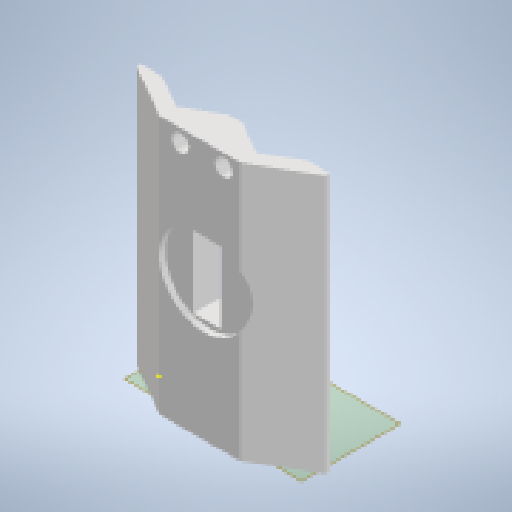
# Autodesk Inventor part: крепеж бок
Saved by Autodesk Inventor 2024.2 (Build 282272000, 272)
## iProperties
Created: 2026-04-23
Part Number: крепеж бок
Material: Типовые
Document SubType Name: Modeling
Designer: katya_notebook
Density: 1 g/cm^3
Appearance: По умолчанию
Author: katya_notebook
Autodesk Inventor part; units mm, degrees
ref_plane "YZ Plane" through (0, 0, 0) normal (1, 0, 0) x (0, 1, 0)
ref_plane "XZ Plane" through (0, 0, 0) normal (0, 1, 0) x (-1, 0, 0)
ref_plane "РабПлоскость1" through (19.6, -8, -11) normal (0, -1, 0) x (-1, 0, 0)
sketch "Эскиз1" plane through (19.6, -8, -11) normal (0, -1, 0) x (-1, 0, 0)
  line L0 (29.4, -5.9741) -> (29.4, 5.9741) projected
  line L1 (28.2551, 5.9741) -> (29.4, 5.9741) projected
  line L2 (28.65, 6.658) -> (28.2551, 5.9741) projected
  line L3 (27.6679, 6.658) -> (28.65, 6.658) projected
  line L4 (21.3321, 10.3161) -> (27.6679, 6.658) projected
  line L5 (21.3321, 10.3161) -> (20.35, 10.3161) projected
  line L6 (20.35, 10.3161) -> (20.5955, 10.7413) projected
  line L7 (20.1474, 11) -> (20.5955, 10.7413) projected
  line L8 (20.1474, 11) -> (19.0526, 11) projected
  line L9 (18.6045, 10.7413) -> (19.0526, 11) projected
  line L10 (18.85, 10.3161) -> (18.6045, 10.7413) projected
  line L11 (17.8679, 10.3161) -> (18.85, 10.3161) projected
  line L12 (11.5321, 6.658) -> (17.8679, 10.3161) projected
  line L13 (11.5321, 6.658) -> (10.55, 6.658) projected
  line L14 (10.55, 6.658) -> (10.9449, 5.9741) projected
  line L15 (8.6551, 5.9741) -> (10.9449, 5.9741) projected
  line L16 (9.05, 6.658) -> (8.6551, 5.9741) projected
  line L17 (8.0679, 6.658) -> (9.05, 6.658) projected
  line L18 (1.7321, 10.3161) -> (8.0679, 6.658) projected
  line L19 (1.7321, 10.3161) -> (0.75, 10.3161) projected
  line L20 (0.75, 10.3161) -> (0.9955, 10.7413) projected
  line L21 (0.5474, 11) -> (0.9955, 10.7413) projected
  line L22 (-0.5474, 11) -> (0.5474, 11) projected
  line L23 (-0.9955, 10.7413) -> (-0.5474, 11) projected
  line L24 (-0.75, 10.3161) -> (-0.9955, 10.7413) projected
  line L25 (-1.7321, 10.3161) -> (-0.75, 10.3161) projected
  line L26 (-8.0679, 6.658) -> (-1.7321, 10.3161) projected
  line L27 (-8.0679, 6.658) -> (-9.05, 6.658) projected
  line L28 (-9.05, 6.658) -> (-8.6551, 5.9741) projected
  line L29 (-8.6551, 5.9741) -> (-9.8, 5.9741) projected
  line L30 (-9.8, -5.9741) -> (-9.8, 5.9741) projected
  line L31 (-8.6551, -5.9741) -> (-9.8, -5.9741) projected
  line L32 (-9.05, -6.658) -> (-8.6551, -5.9741) projected
  line L33 (-8.0679, -6.658) -> (-9.05, -6.658) projected
  line L34 (-1.7321, -10.3161) -> (-8.0679, -6.658) projected
  line L35 (-1.7321, -10.3161) -> (-0.75, -10.3161) projected
  line L36 (-0.75, -10.3161) -> (-0.9955, -10.7413) projected
  line L37 (-0.5474, -11) -> (-0.9955, -10.7413) projected
  line L38 (-0.5474, -11) -> (0.5474, -11) projected
  line L39 (0.9955, -10.7413) -> (0.5474, -11) projected
  line L40 (0.75, -10.3161) -> (0.9955, -10.7413) projected
  line L41 (1.7321, -10.3161) -> (0.75, -10.3161) projected
  line L42 (8.0679, -6.658) -> (1.7321, -10.3161) projected
  line L43 (8.0679, -6.658) -> (9.05, -6.658) projected
  line L44 (9.05, -6.658) -> (8.6551, -5.9741) projected
  line L45 (8.6551, -5.9741) -> (10.9449, -5.9741) projected
  line L46 (10.55, -6.658) -> (10.9449, -5.9741) projected
  line L47 (11.5321, -6.658) -> (10.55, -6.658) projected
  line L48 (17.8679, -10.3161) -> (11.5321, -6.658) projected
  line L49 (17.8679, -10.3161) -> (18.85, -10.3161) projected
  line L50 (18.85, -10.3161) -> (18.6045, -10.7413) projected
  line L51 (19.0526, -11) -> (18.6045, -10.7413) projected
  line L52 (19.0526, -11) -> (20.1474, -11) projected
  line L53 (20.5955, -10.7413) -> (20.1474, -11) projected
  line L54 (20.35, -10.3161) -> (20.5955, -10.7413) projected
  line L55 (21.3321, -10.3161) -> (20.35, -10.3161) projected
  line L56 (27.6679, -6.658) -> (21.3321, -10.3161) projected
  line L57 (27.6679, -6.658) -> (28.65, -6.658) projected
  line L58 (28.65, -6.658) -> (28.2551, -5.9741) projected
  line L59 (28.2551, -5.9741) -> (29.4, -5.9741) projected
  circle A0 centre (0, 0) radius 8.1 projected
  circle A1 centre (19.6, 0) radius 8.1 projected
  line L60 (32.9, 3.6373) -> (42.7, 9.2953) projected
  line L61 (42.7, 9.2953) -> (42.7, 24.6529) projected
  line L62 (42.7, 24.6529) -> (29.4, 32.3316) projected
  line L63 (29.4, 32.3316) -> (19.6, 26.6736) projected
  line L64 (19.6, 26.6736) -> (9.8, 32.3316) projected
  line L65 (9.8, 32.3316) -> (0, 26.6736) projected
  line L66 (0, 26.6736) -> (-9.8, 32.3316) projected
  line L67 (-9.8, 32.3316) -> (-23.1, 24.6529) projected
  line L68 (-23.1, 24.6529) -> (-23.1, 9.2953) projected
  line L69 (-23.1, 9.2953) -> (-13.3, 3.6373) projected
  line L70 (-13.3, 3.6373) -> (-13.3, -7.6788) projected
  line L71 (29.4, -5.9741) -> (28.2551, -5.9741) projected
  line L72 (28.2551, -5.9741) -> (28.65, -6.658) projected
  line L73 (28.65, -6.658) -> (27.6679, -6.658) projected
  line L74 (27.6679, -6.658) -> (21.3321, -10.3161) projected
  line L75 (17.8679, -10.3161) -> (11.5321, -6.658) projected
  line L76 (11.5321, -6.658) -> (10.55, -6.658) projected
  line L77 (10.55, -6.658) -> (10.9449, -5.9741) projected
  line L78 (10.9449, -5.9741) -> (8.6551, -5.9741) projected
  line L79 (8.6551, -5.9741) -> (9.05, -6.658) projected
  line L80 (9.05, -6.658) -> (8.0679, -6.658) projected
  line L81 (8.0679, -6.658) -> (1.7321, -10.3161) projected
  line L82 (-1.7321, -10.3161) -> (-8.0679, -6.658) projected
  line L83 (-8.0679, -6.658) -> (-9.05, -6.658) projected
  line L84 (-9.05, -6.658) -> (-8.6551, -5.9741) projected
  line L85 (-8.6551, -5.9741) -> (-9.8, -5.9741) projected
  line L86 (-9.8, -5.9741) -> (-9.8, 5.9741) projected
  line L87 (-9.8, 5.9741) -> (-10.3474, 5.9741) projected
  line L88 (-10.3474, 5.9741) -> (-10.7955, 6.2328) projected
  line L89 (-10.7955, 6.2328) -> (-10.55, 6.658) projected
  line L90 (-10.55, 6.658) -> (-11.5321, 6.658) projected
  line L91 (-11.5321, 6.658) -> (-17.8679, 10.3161) projected
  line L92 (-17.8679, 10.3161) -> (-18.85, 10.3161) projected
  line L93 (-18.85, 10.3161) -> (-18.4551, 11) projected
  line L94 (-18.4551, 11) -> (-19.6, 11) projected
  line L95 (-19.6, 11) -> (-19.6, 22.9482) projected
  line L96 (-19.6, 22.9482) -> (-18.4551, 22.9482) projected
  line L97 (-18.4551, 22.9482) -> (-18.85, 23.6321) projected
  line L98 (-18.85, 23.6321) -> (-17.8679, 23.6321) projected
  line L99 (-17.8679, 23.6321) -> (-11.5321, 27.2902) projected
  line L100 (-11.5321, 27.2902) -> (-10.55, 27.2902) projected
  line L101 (-10.55, 27.2902) -> (-10.7955, 27.7154) projected
  line L102 (-10.7955, 27.7154) -> (-10.3474, 27.9741) projected
  line L103 (-10.3474, 27.9741) -> (-9.2526, 27.9741) projected
  line L104 (-9.2526, 27.9741) -> (-8.8045, 27.7154) projected
  line L105 (-8.8045, 27.7154) -> (-9.05, 27.2902) projected
  line L106 (-9.05, 27.2902) -> (-8.0679, 27.2902) projected
  line L107 (-8.0679, 27.2902) -> (-1.7321, 23.6321) projected
  line L108 (-1.7321, 23.6321) -> (-0.75, 23.6321) projected
  line L109 (-0.75, 23.6321) -> (-1.1449, 22.9482) projected
  line L110 (-1.1449, 22.9482) -> (1.1449, 22.9482) projected
  line L111 (1.1449, 22.9482) -> (0.75, 23.6321) projected
  line L112 (0.75, 23.6321) -> (1.7321, 23.6321) projected
  line L113 (1.7321, 23.6321) -> (8.0679, 27.2902) projected
  line L114 (8.0679, 27.2902) -> (9.05, 27.2902) projected
  line L115 (9.05, 27.2902) -> (8.8045, 27.7154) projected
  line L116 (8.8045, 27.7154) -> (9.2526, 27.9741) projected
  line L117 (9.2526, 27.9741) -> (10.3474, 27.9741) projected
  line L118 (10.3474, 27.9741) -> (10.7955, 27.7154) projected
  line L119 (10.7955, 27.7154) -> (10.55, 27.2902) projected
  line L120 (10.55, 27.2902) -> (11.5321, 27.2902) projected
  line L121 (11.5321, 27.2902) -> (17.8679, 23.6321) projected
  line L122 (17.8679, 23.6321) -> (18.85, 23.6321) projected
  line L123 (18.85, 23.6321) -> (18.4551, 22.9482) projected
  line L124 (18.4551, 22.9482) -> (20.7449, 22.9482) projected
  line L125 (20.7449, 22.9482) -> (20.35, 23.6321) projected
  line L126 (20.35, 23.6321) -> (21.3321, 23.6321) projected
  line L127 (21.3321, 23.6321) -> (27.6679, 27.2902) projected
  line L128 (27.6679, 27.2902) -> (28.65, 27.2902) projected
  line L129 (28.65, 27.2902) -> (28.4045, 27.7154) projected
  line L130 (28.4045, 27.7154) -> (28.8526, 27.9741) projected
  line L131 (28.8526, 27.9741) -> (29.9474, 27.9741) projected
  line L132 (29.9474, 27.9741) -> (30.3955, 27.7154) projected
  line L133 (30.3955, 27.7154) -> (30.15, 27.2902) projected
  line L134 (30.15, 27.2902) -> (31.1321, 27.2902) projected
  line L135 (31.1321, 27.2902) -> (37.4679, 23.6321) projected
  line L136 (37.4679, 23.6321) -> (38.45, 23.6321) projected
  line L137 (38.45, 23.6321) -> (38.0551, 22.9482) projected
  line L138 (38.0551, 22.9482) -> (39.2, 22.9482) projected
  line L139 (39.2, 22.9482) -> (39.2, 11) projected
  line L140 (39.2, 11) -> (38.0551, 11) projected
  line L141 (38.0551, 11) -> (38.45, 10.3161) projected
  line L142 (38.45, 10.3161) -> (37.4679, 10.3161) projected
  line L143 (37.4679, 10.3161) -> (31.1321, 6.658) projected
  line L144 (31.1321, 6.658) -> (30.15, 6.658) projected
  line L145 (30.15, 6.658) -> (30.3955, 6.2328) projected
  line L146 (30.3955, 6.2328) -> (29.9474, 5.9741) projected
  line L147 (29.9474, 5.9741) -> (29.4, 5.9741) projected
  line L148 (29.4, 5.9741) -> (29.4, -5.9741) projected
  line L149 (-13.3, -7.6788) -> (0, -15.3575) projected
  line L150 (0, -15.3575) -> (9.8, -9.6995) projected
  line L151 (9.8, -9.6995) -> (19.6, -15.3575) projected
  line L152 (19.6, -15.3575) -> (32.9, -7.6788) projected
  line L153 (32.9, -7.6788) -> (32.9, 3.6373) projected
  line L154 (21.3321, -10.3161) -> (20.35, -10.3161) projected
  line L155 (20.35, -10.3161) -> (20.5955, -10.7413) projected
  line L156 (20.5955, -10.7413) -> (20.1474, -11) projected
  line L157 (20.1474, -11) -> (19.0526, -11) projected
  line L158 (19.0526, -11) -> (18.6045, -10.7413) projected
  line L159 (18.6045, -10.7413) -> (18.85, -10.3161) projected
  line L160 (18.85, -10.3161) -> (17.8679, -10.3161) projected
  line L161 (1.7321, -10.3161) -> (0.75, -10.3161) projected
  line L162 (0.75, -10.3161) -> (0.9955, -10.7413) projected
  line L163 (0.9955, -10.7413) -> (0.5474, -11) projected
  line L164 (0.5474, -11) -> (-0.5474, -11) projected
  line L165 (-0.5474, -11) -> (-0.9955, -10.7413) projected
  line L166 (-0.9955, -10.7413) -> (-0.75, -10.3161) projected
  line L167 (-0.75, -10.3161) -> (-1.7321, -10.3161) projected
  line L168 (32.9, -5.9741) -> (29.4, -5.9741)
  line L169 (-9.8, -5.9741) -> (-13.3, -5.9741)
  line L170 (19.6, -15.3575) -> (0, -15.3575)
  point P0 (19.6, -11)
  constraints: 6 end point, 2 perpendicular, 2 point on line, 1 horizontal
ref_plane "РабПлоскость2" through (-38.0502, 55.1, -60.2624) normal (0, -1, 0) x (1, 0, 0)
extrude "Выдавливание1" add sketch "Эскиз1" against normal up to surface (63.1 mm away) contours L168 L153 L152 L151 L150 L149 L70 L169 L31 L32 L33 L34 L35 L36 L37 L38 L39 L40 L41 L42 L43 L44 L45 L46 L47 L48 L49 L50 L51 L52 L53 L54 L55 L56 L57 L58 L59 | L170 L150 L151
sketch "Эскиз2" plane through (0, -8, 4.3575) normal (0, 0, 1) x (1, 0, 0)
  circle A0 centre (10.0964, 32.8819) radius 10.85 projected
  spline S0 degree 3 poles (1.2199, 29.8332) (1.2264, 29.8391) (1.2399, 29.8514) (1.2666, 29.8618) (1.2971, 29.8679) (1.3188, 29.8674) (1.3303, 29.8671) knots 0 0 0 0 0.219432 0.455746 0.710361 1 1 1 1 projected
  line L0 (1.3303, 29.8671) -> (4.8998, 29.6603) projected
  line L1 (4.8998, 29.6603) -> (4.9412, 30.3747) projected
  spline S1 degree 3 poles (4.9412, 30.3747) (4.9436, 30.3952) (4.948, 30.4343) (4.9731, 30.4645) (4.9851, 30.4789) knots 0 0 0 0 0.523055 1 1 1 1 projected
  spline S2 degree 3 poles (4.9851, 30.4789) (5.0002, 30.4888) (5.0301, 30.5084) (5.0658, 30.5096) (5.0835, 30.5102) knots 0 0 0 0 0.505194 1 1 1 1 projected
  spline S3 degree 3 poles (5.0835, 30.5102) (5.0953, 30.507) (5.1242, 30.4991) (5.1574, 30.4755) (5.186, 30.4505) (5.2006, 30.4236) (5.2097, 30.3936) (5.2095, 30.3722) (5.2093, 30.3609) knots 0 0 0 0 0.170693 0.418909 0.563896 0.700202 0.841955 1 1 1 1 projected
  line L2 (5.2093, 30.3609) -> (5.1108, 28.6607) projected
  spline S4 degree 3 poles (5.1108, 28.6607) (5.1075, 28.6439) (5.1004, 28.6081) (5.064, 28.5657) (5.0204, 28.5312) (4.985, 28.5283) (4.9686, 28.5269) knots 0 0 0 0 0.239185 0.507115 0.772399 1 1 1 1 projected
  spline S5 degree 3 poles (4.9686, 28.5269) (4.9527, 28.5298) (4.9195, 28.5357) (4.8843, 28.5622) (4.8611, 28.5897) (4.8491, 28.6156) (4.842, 28.6452) (4.8426, 28.6661) (4.8429, 28.6771) knots 0 0 0 0 0.219722 0.460095 0.585443 0.71296 0.849405 1 1 1 1 projected
  line L3 (4.8429, 28.6771) -> (4.8843, 29.3923) projected
  line L4 (4.8843, 29.3923) -> (1.3148, 29.5991) projected
  spline S6 degree 3 poles (1.3148, 29.5991) (1.2937, 29.6014) (1.254, 29.6057) (1.2233, 29.6311) (1.2089, 29.6431) knots 0 0 0 0 0.529822 1 1 1 1 projected
  spline S7 degree 3 poles (1.2089, 29.6431) (1.1996, 29.6574) (1.1802, 29.6872) (1.1802, 29.7228) (1.1802, 29.7414) knots 0 0 0 0 0.479535 1 1 1 1 projected
  spline S8 degree 3 poles (1.1802, 29.7414) (1.1812, 29.7464) (1.1836, 29.7582) (1.1913, 29.7787) (1.2037, 29.8042) (1.2142, 29.8229) (1.2199, 29.8332) knots 0 0 0 0 0.152278 0.360896 0.649123 1 1 1 1 projected
  line L5 (5.314, 32.1682) -> (5.2899, 31.752) projected
  spline S9 degree 3 poles (5.2899, 31.752) (5.2876, 31.7272) (5.2829, 31.6758) (5.2703, 31.5966) (5.2484, 31.514) (5.2231, 31.428) (5.1921, 31.3426) (5.1551, 31.2607) (5.1134, 31.1842) (5.0808, 31.137) (5.0647, 31.1138) knots 0 0 0 0 0.109156 0.226197 0.350912 0.483159 0.618823 0.74875 0.876439 1 1 1 1 projected
  spline S10 degree 3 poles (5.0647, 31.1138) (5.0604, 31.1082) (5.0508, 31.0957) (5.0277, 31.0797) (4.9933, 31.0643) (4.9651, 31.0584) (4.9487, 31.055) knots 0 0 0 0 0.157275 0.353812 0.623959 1 1 1 1 projected
  spline S11 degree 3 poles (4.9487, 31.055) (4.931, 31.0577) (4.8944, 31.0635) (4.8502, 31.0969) (4.8148, 31.1372) (4.811, 31.1704) (4.8092, 31.1857) knots 0 0 0 0 0.254223 0.52772 0.782584 1 1 1 1 projected
  line L6 (4.8092, 31.1857) -> (4.839, 31.2655) projected
  spline S12 degree 3 poles (4.839, 31.2655) (4.8649, 31.302) (4.9161, 31.3743) (4.9704, 31.4963) (5.009, 31.625) (5.0173, 31.7147) (5.0215, 31.76) knots 0 0 0 0 0.250207 0.496054 0.745305 1 1 1 1 projected
  line L7 (5.0215, 31.76) -> (5.0462, 32.1871) projected
  spline S13 degree 3 poles (5.0462, 32.1871) (5.0465, 32.2279) (5.047, 32.3069) (5.0221, 32.4217) (4.9727, 32.5253) (4.9041, 32.6172) (4.8204, 32.6936) (4.7258, 32.7518) (4.6219, 32.7904) (4.5485, 32.7982) (4.5113, 32.8021) knots 0 0 0 0 0.134588 0.260434 0.384536 0.51119 0.637382 0.756913 0.876544 1 1 1 1 projected
  line L8 (4.5113, 32.8021) -> (4.3969, 32.8004) projected
  line L9 (4.3969, 32.8004) -> (4.3418, 32.7918) projected
  line L10 (4.3418, 32.7918) -> (4.2895, 32.7747) projected
  spline S14 degree 3 poles (4.2895, 32.7747) (4.2759, 32.7681) (4.2464, 32.7539) (4.201, 32.7264) (4.1502, 32.6923) (4.1153, 32.6662) (4.0967, 32.6522) knots 0 0 0 0 0.198705 0.428492 0.695375 1 1 1 1 projected
  line L11 (4.0967, 32.6522) -> (2.7508, 31.4386) projected
  spline S15 degree 3 poles (2.7508, 31.4386) (2.7287, 31.4196) (2.6853, 31.3821) (2.6147, 31.3335) (2.5398, 31.2938) (2.4871, 31.2738) (2.4608, 31.2638) knots 0 0 0 0 0.25594 0.505009 0.752321 1 1 1 1 projected
  line L12 (2.4608, 31.2638) -> (2.3941, 31.2441) projected
  line L13 (2.3941, 31.2441) -> (2.2844, 31.2219) projected
  line L14 (2.2844, 31.2219) -> (2.2184, 31.214) projected
  line L15 (2.2184, 31.214) -> (2.1355, 31.2188) projected
  spline S16 degree 3 poles (2.1355, 31.2188) (2.1073, 31.221) (2.0518, 31.2253) (1.9706, 31.2414) (1.8929, 31.264) (1.8193, 31.2949) (1.7487, 31.3318) (1.6814, 31.3759) (1.6185, 31.428) (1.5798, 31.4669) (1.5603, 31.4866) knots 0 0 0 0 0.130274 0.256409 0.380833 0.502298 0.624003 0.747576 0.872087 1 1 1 1 projected
  spline S17 degree 3 poles (1.5603, 31.4866) (1.5403, 31.5086) (1.501, 31.552) (1.4514, 31.6239) (1.409, 31.6982) (1.3765, 31.777) (1.3515, 31.8588) (1.3368, 31.9447) (1.3286, 32.0337) (1.3307, 32.0942) (1.3317, 32.125) knots 0 0 0 0 0.127376 0.251339 0.373922 0.494219 0.616919 0.74041 0.867775 1 1 1 1 projected
  line L16 (1.3317, 32.125) -> (1.3558, 32.5404) projected
  spline S18 degree 3 poles (1.3558, 32.5404) (1.3581, 32.57) (1.3627, 32.6288) (1.3785, 32.7152) (1.3986, 32.7994) (1.4276, 32.8801) (1.4612, 32.9589) (1.503, 33.0341) (1.5498, 33.1077) (1.5861, 33.1534) (1.6044, 33.1765) knots 0 0 0 0 0.128087 0.254502 0.3786 0.501671 0.623923 0.748156 0.873068 1 1 1 1 projected
  line L17 (1.6044, 33.1765) -> (1.6608, 33.2219) projected
  line L18 (1.6608, 33.2219) -> (1.7278, 33.2323) projected
  spline S19 degree 3 poles (1.7278, 33.2323) (1.7436, 33.2293) (1.7788, 33.2226) (1.8172, 33.1955) (1.8457, 33.1692) (1.862, 33.1468) (1.8715, 33.123) (1.872, 33.1067) (1.8722, 33.0988) knots 0 0 0 0 0.225013 0.500357 0.645758 0.771988 0.888482 1 1 1 1 projected
  line L19 (1.8722, 33.0988) -> (1.8363, 33.0168) projected
  spline S20 degree 3 poles (1.8363, 33.0168) (1.8059, 32.9802) (1.7465, 32.909) (1.6822, 32.7873) (1.6385, 32.66) (1.6288, 32.5716) (1.6239, 32.5274) knots 0 0 0 0 0.262033 0.510647 0.755153 1 1 1 1 projected
  line L20 (1.6239, 32.5274) -> (1.5994, 32.1045) projected
  spline S21 degree 3 poles (1.5994, 32.1045) (1.5993, 32.0662) (1.5991, 31.9907) (1.6258, 31.8801) (1.6754, 31.7771) (1.7439, 31.6831) (1.827, 31.6017) (1.9225, 31.5408) (2.0268, 31.4999) (2.1004, 31.4917) (2.1376, 31.4876) knots 0 0 0 0 0.126552 0.249346 0.372878 0.503227 0.632635 0.755805 0.876214 1 1 1 1 projected
  line L21 (2.1376, 31.4876) -> (2.2344, 31.4904) projected
  spline S22 degree 3 poles (2.2344, 31.4904) (2.2424, 31.4911) (2.2593, 31.4927) (2.2852, 31.4995) (2.3126, 31.5062) (2.3305, 31.5129) (2.3393, 31.5162) knots 0 0 0 0 0.220277 0.47027 0.739664 1 1 1 1 projected
  spline S23 degree 3 poles (2.3393, 31.5162) (2.3561, 31.5216) (2.3912, 31.5327) (2.4427, 31.5592) (2.4967, 31.5921) (2.5308, 31.6198) (2.5487, 31.6344) knots 0 0 0 0 0.217508 0.45648 0.715095 1 1 1 1 projected
  line L22 (2.5487, 31.6344) -> (3.8947, 32.8496) projected
  spline S24 degree 3 poles (3.8947, 32.8496) (3.9135, 32.8658) (3.9528, 32.8998) (4.0224, 32.9431) (4.0991, 32.9892) (4.1556, 33.0157) (4.1849, 33.0295) knots 0 0 0 0 0.216591 0.454587 0.716038 1 1 1 1 projected
  spline S25 degree 3 poles (4.1849, 33.0295) (4.2113, 33.037) (4.2639, 33.0522) (4.3449, 33.067) (4.4272, 33.0731) (4.4823, 33.0718) (4.5101, 33.0711) knots 0 0 0 0 0.249589 0.498449 0.747622 1 1 1 1 projected
  spline S26 degree 3 poles (4.5101, 33.0711) (4.5383, 33.0689) (4.5938, 33.0646) (4.675, 33.0485) (4.7526, 33.0259) (4.8263, 32.995) (4.8966, 32.958) (4.9644, 32.915) (5.0271, 32.8627) (5.0658, 32.8238) (5.0853, 32.8042) knots 0 0 0 0 0.130358 0.256573 0.381077 0.50262 0.624402 0.747414 0.872005 1 1 1 1 projected
  spline S27 degree 3 poles (5.0853, 32.8042) (5.1053, 32.7822) (5.1447, 32.7388) (5.1939, 32.667) (5.2369, 32.5933) (5.2689, 32.5147) (5.2944, 32.4334) (5.3089, 32.3477) (5.317, 32.259) (5.3151, 32.1988) (5.314, 32.1682) knots 0 0 0 0 0.127803 0.252181 0.37416 0.49486 0.61684 0.740744 0.868535 1 1 1 1 projected
  spline S28 degree 3 poles (3.6331, 34.2513) (3.6171, 34.2541) (3.5836, 34.26) (3.549, 34.2875) (3.5256, 34.3149) (3.5136, 34.3409) (3.5065, 34.3704) (3.5071, 34.3913) (3.5074, 34.4023) knots 0 0 0 0 0.219271 0.461203 0.586294 0.713549 0.849714 1 1 1 1 projected
  line L23 (3.5074, 34.4023) -> (3.5487, 35.1167) projected
  line L24 (3.5487, 35.1167) -> (1.7799, 35.2192) projected
  line L25 (1.7799, 35.2192) -> (1.7054, 33.9336) projected
  spline S29 degree 3 poles (1.7054, 33.9336) (1.7021, 33.9168) (1.695, 33.8811) (1.6586, 33.8386) (1.6149, 33.8043) (1.5795, 33.8007) (1.5632, 33.799) knots 0 0 0 0 0.238964 0.506645 0.771683 1 1 1 1 projected
  spline S30 degree 3 poles (1.5632, 33.799) (1.5473, 33.8019) (1.514, 33.8078) (1.4789, 33.8343) (1.4556, 33.8618) (1.4436, 33.8877) (1.4366, 33.917) (1.4371, 33.9376) (1.4374, 33.9483) knots 0 0 0 0 0.220569 0.461868 0.587699 0.715707 0.852678 1 1 1 1 projected
  line L26 (1.4374, 33.9483) -> (1.5192, 35.3612) projected
  spline S31 degree 3 poles (1.5192, 35.3612) (1.5219, 35.3821) (1.5267, 35.4202) (1.5572, 35.4694) (1.6096, 35.494) (1.6479, 35.4943) (1.669, 35.4946) knots 0 0 0 0 0.274617 0.5 0.725383 1 1 1 1 projected
  line L27 (1.669, 35.4946) -> (5.3524, 35.2811) projected
  spline S32 degree 3 poles (5.3524, 35.2811) (5.3733, 35.2785) (5.4113, 35.2737) (5.4605, 35.2432) (5.4851, 35.1908) (5.4855, 35.1525) (5.4857, 35.1314) knots 0 0 0 0 0.274617 0.5 0.725383 1 1 1 1 projected
  line L28 (5.4857, 35.1314) -> (5.4039, 33.7185) projected
  spline S33 degree 3 poles (5.4039, 33.7185) (5.4005, 33.7017) (5.3934, 33.6659) (5.3571, 33.6235) (5.3134, 33.589) (5.278, 33.5861) (5.2617, 33.5847) knots 0 0 0 0 0.239185 0.507115 0.772399 1 1 1 1 projected
  spline S34 degree 3 poles (5.2617, 33.5847) (5.2457, 33.5875) (5.2122, 33.5934) (5.1776, 33.6208) (5.1542, 33.6483) (5.1422, 33.6742) (5.1352, 33.7035) (5.1356, 33.7242) (5.1359, 33.7349) knots 0 0 0 0 0.220114 0.462976 0.588548 0.716293 0.852982 1 1 1 1 projected
  line L29 (5.1359, 33.7349) -> (5.2104, 35.0205) projected
  line L30 (5.2104, 35.0205) -> (3.8168, 35.1012) projected
  line L31 (3.8168, 35.1012) -> (3.7754, 34.3868) projected
  spline S35 degree 3 poles (3.7754, 34.3868) (3.772, 34.3697) (3.7651, 34.3336) (3.7285, 34.2909) (3.6848, 34.2566) (3.6494, 34.253) (3.6331, 34.2513) knots 0 0 0 0 0.241893 0.508544 0.772562 1 1 1 1 projected
  spline S36 degree 3 poles (1.6423, 37.123) (1.6488, 37.1289) (1.6622, 37.1412) (1.689, 37.1516) (1.7195, 37.1577) (1.7411, 37.1572) (1.7527, 37.1569) knots 0 0 0 0 0.219432 0.455746 0.710361 1 1 1 1 projected
  line L32 (1.7527, 37.1569) -> (5.3222, 36.9501) projected
  line L33 (5.3222, 36.9501) -> (5.3636, 37.6645) projected
  spline S37 degree 3 poles (5.3636, 37.6645) (5.3659, 37.685) (5.3704, 37.7241) (5.3955, 37.7543) (5.4074, 37.7687) knots 0 0 0 0 0.523055 1 1 1 1 projected
  spline S38 degree 3 poles (5.4074, 37.7687) (5.4225, 37.7786) (5.4525, 37.7982) (5.4882, 37.7994) (5.5059, 37.8) knots 0 0 0 0 0.505194 1 1 1 1 projected
  spline S39 degree 3 poles (5.5059, 37.8) (5.5177, 37.7967) (5.5466, 37.7889) (5.5798, 37.7652) (5.6084, 37.7402) (5.623, 37.7134) (5.6321, 37.6834) (5.6318, 37.662) (5.6317, 37.6507) knots 0 0 0 0 0.170693 0.418909 0.563896 0.700202 0.841955 1 1 1 1 projected
  line L34 (5.6317, 37.6507) -> (5.5332, 35.9505) projected
  spline S40 degree 3 poles (5.5332, 35.9505) (5.5298, 35.9336) (5.5228, 35.8979) (5.4864, 35.8555) (5.4427, 35.8209) (5.4073, 35.8181) (5.391, 35.8167) knots 0 0 0 0 0.239185 0.507115 0.772399 1 1 1 1 projected
  spline S41 degree 3 poles (5.391, 35.8167) (5.3751, 35.8196) (5.3418, 35.8255) (5.3067, 35.852) (5.2834, 35.8795) (5.2714, 35.9054) (5.2644, 35.935) (5.2649, 35.9559) (5.2652, 35.9669) knots 0 0 0 0 0.219722 0.460095 0.585443 0.71296 0.849405 1 1 1 1 projected
  line L35 (5.2652, 35.9669) -> (5.3067, 36.6821) projected
  line L36 (5.3067, 36.6821) -> (1.7371, 36.8889) projected
  spline S42 degree 3 poles (1.7371, 36.8889) (1.7161, 36.8912) (1.6764, 36.8955) (1.6457, 36.9209) (1.6313, 36.9329) knots 0 0 0 0 0.529822 1 1 1 1 projected
  spline S43 degree 3 poles (1.6313, 36.9329) (1.622, 36.9472) (1.6025, 36.977) (1.6025, 37.0126) (1.6025, 37.0312) knots 0 0 0 0 0.479535 1 1 1 1 projected
  spline S44 degree 3 poles (1.6025, 37.0312) (1.6035, 37.0362) (1.606, 37.048) (1.6136, 37.0685) (1.6261, 37.094) (1.6366, 37.1127) (1.6423, 37.123) knots 0 0 0 0 0.152278 0.360896 0.649123 1 1 1 1 projected
  arc A1 (13.962, 34.3771) -> (13.7634, 30.9503) centre (10.0964, 32.8819) ccw projected
  line L37 (13.962, 34.3771) -> (13.2158, 34.0885) projected
  arc A2 (13.2158, 34.0885) -> (13.0556, 31.3231) centre (10.0964, 32.8819) ccw projected
  line L38 (13.0556, 31.3231) -> (13.7634, 30.9503) projected
  line L39 (14.9235, 33.0029) -> (12.2087, 33.1602) projected
  line L40 (14.9235, 33.0029) -> (14.8772, 32.2042) projected
  line L41 (14.8772, 32.2042) -> (12.1624, 32.3615) projected
  line L42 (12.1624, 32.3615) -> (12.2087, 33.1602) projected
  line L43 (13.5198, 41.5398) -> (6.7574, 41.5398)
  line L44 (6.7574, 41.5398) -> (6.7574, 24.0382)
  line L45 (6.7574, 24.0382) -> (13.5198, 24.0382)
  line L46 (13.5198, 24.0382) -> (13.5198, 41.5398)
  point P0 (0, 8)
  constraints: 8 end point, 2 parallel, 1 horizontal, 1 perpendicular
extrude "Выдавливание2" cut sketch "Эскиз2" against normal blind 10 contours L46 L37 A2 L44 A1 | A1 L44 L43 L46 | L46 L39 L42 L41 L38 A2 L44 L37 | L46 L41 L42 L39 | L44 A2 L38 L46 A1 | A1 L46 L45 L44
sketch "Эскиз3" plane through (0, -8, 4.3575) normal (0, 0, 1) x (1, 0, 0)
  circle A0 centre (10.8015, 33.6616) radius 10.85 projected
  point P0 (0, 8)
extrude "Выдавливание3" cut sketch "Эскиз3" against normal blind 1.5
sketch "Эскиз4" plane through (0, 55.1, 4.3575) normal (0, 0, 1) x (1, 0, 0)
  point P0 (0, -55.1)
sketch "Эскиз5" plane through (0, 55.1, 4.3575) normal (0, 0, 1) x (1, 0, 0)
  ellipse E0 centre (15.6791, -3.0669) end of major axis (15.6791, -1.0669) minor radius 2 projected
  ellipse E1 centre (4.9612, -3.0669) end of major axis (4.9612, -1.0669) minor radius 2 projected
  circle A0 centre (15.6791, -3.0669) radius 2.1
  circle A1 centre (4.9612, -3.0669) radius 2.1
  point P0 (0, -55.1)
  dimension "d10" = 4.2
  dimension "d11" = 4.2
  constraints: 2 centre point, 2 coincident, 2 other
  measures "d10" diameter of A0
  measures "d11" diameter of A1
extrude "Выдавливание4" cut sketch "Эскиз5" against normal blind 5 contours E0 | E1 | A0 | A1
sketch "Эскиз6" plane through (0, 55.1, 4.3575) normal (0, 1, 0) x (1, 0, 0)
  line L0 (-8.6551, 9.3834) -> (-13.3, 9.3834) projected
  line L1 (-13.3, 9.3834) -> (-13.3, 7.6788) projected
  line L2 (-13.3, 7.6788) -> (0, 0) projected
  line L3 (0, 0) -> (19.6, 0) projected
  line L4 (19.6, 0) -> (32.9, 7.6788) projected
  line L5 (32.9, 7.6788) -> (32.9, 9.3834) projected
  line L6 (32.9, 9.3834) -> (28.2551, 9.3834) projected
  line L7 (28.2551, 9.3834) -> (28.65, 8.6995) projected
  line L8 (28.65, 8.6995) -> (27.6679, 8.6995) projected
  line L9 (27.6679, 8.6995) -> (21.3321, 5.0415) projected
  line L10 (21.3321, 5.0415) -> (20.35, 5.0415) projected
  line L11 (20.35, 5.0415) -> (20.5955, 4.6162) projected
  line L12 (20.5955, 4.6162) -> (20.1474, 4.3575) projected
  line L13 (20.1474, 4.3575) -> (19.0526, 4.3575) projected
  line L14 (19.0526, 4.3575) -> (18.6045, 4.6162) projected
  line L15 (18.6045, 4.6162) -> (18.85, 5.0415) projected
  line L16 (18.85, 5.0415) -> (17.8679, 5.0415) projected
  line L17 (17.8679, 5.0415) -> (11.5321, 8.6995) projected
  line L18 (11.5321, 8.6995) -> (10.55, 8.6995) projected
  line L19 (10.55, 8.6995) -> (10.9449, 9.3834) projected
  line L20 (10.9449, 9.3834) -> (8.6551, 9.3834) projected
  line L21 (8.6551, 9.3834) -> (9.05, 8.6995) projected
  line L22 (9.05, 8.6995) -> (8.0679, 8.6995) projected
  line L23 (8.0679, 8.6995) -> (1.7321, 5.0415) projected
  line L24 (1.7321, 5.0415) -> (0.75, 5.0415) projected
  line L25 (0.75, 5.0415) -> (0.9955, 4.6162) projected
  line L26 (0.9955, 4.6162) -> (0.5474, 4.3575) projected
  line L27 (0.5474, 4.3575) -> (-0.5474, 4.3575) projected
  line L28 (-0.5474, 4.3575) -> (-0.9955, 4.6162) projected
  line L29 (-0.9955, 4.6162) -> (-0.75, 5.0415) projected
  line L30 (-0.75, 5.0415) -> (-1.7321, 5.0415) projected
  line L31 (-1.7321, 5.0415) -> (-8.0679, 8.6995) projected
  line L32 (-8.0679, 8.6995) -> (-9.05, 8.6995) projected
  line L33 (-9.05, 8.6995) -> (-8.6551, 9.3834) projected
  circle A0 centre (0, 15.3575) radius 8.1 projected
  line L34 (-0.9955, 4.6162) -> (3.0148, 2.3009)
  line L35 (-0.9955, 4.6162) -> (-14.4085, 12.3602)
  line L36 (-1.543, 3.1506) -> (10.7474, 10.2465)
  line L37 (19.6, 4.0415) -> (9.8, 9.6995) projected
  line L38 (29.4, 9.6995) -> (19.6, 4.0415) projected
  line L39 (8.0679, 8.6995) -> (11.5321, 8.6995)
  line L40 (-9.05, 8.6995) -> (-13.3, 8.6995)
  line L41 (28.65, 8.6995) -> (32.9, 8.6995)
  point P0 (0, 4.3575)
  point P1 (10.55, 8.6995)
  point P2 (0.9955, 4.6162)
  point P3 (0, 4.0415)
  constraints: 12 end point, 4 point on line, 1 collinear, 1 perpendicular
extrude "Выдавливание5" cut sketch "Эскиз6" against normal up to surface (63.1 mm away) contours L33 L35 L0 | L35 L33 L40 L1 L0 | L30 L29 L35 | L27 L36 L34 | L25 L24 L36 | L41 L7 L38 L6 L5 | L38 L7 L6 | L21 L36 L20 L37 L19 L39 | L21 L20 L36 | L38 L11 L10 | L37 L20 L19 | L38 L37 L13 | L16 L15 L37
sketch "Эскиз7" plane through (19.6, -8, -11) normal (0, -1, 0) x (1, 0, 0)
  line L0 (-6.0802, 13.8575) -> (-6.0802, 7.8057) projected
  line L1 (-6.0802, 12.4575) -> (-18.1272, 12.4575)
  circle A0 centre (-6.0802, 12.4575) radius 2.1
  line L2 (-6.0209, 10.3575) -> (-1.8209, 10.3575) projected
  circle A1 centre (-13.52, 12.4575) radius 2.1
  line L3 (-11.5321, 6.658) -> (-8.0679, 6.658) projected
  point P0 (-19.6, 11)
  point P1 (-9.8, 6.658)
  dimension "d14" = 4.2
  dimension "d15" = 4.2
  dimension "d17" = 3.72
  constraints: 2 centre point, 2 end point, 2 point on line, 1 coincident, 1 horizontal, 1 midpoint, 1 tangent
  measures "d14" diameter of A0
  measures "d15" diameter of A1
  measures "d17" horizontal distance of point (-9.8, 6.658) A1.centre
extrude "Выдавливание6" cut sketch "Эскиз7" against normal blind 3
